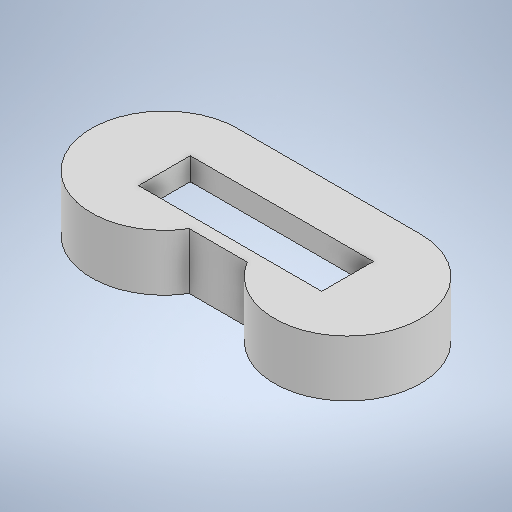
# Autodesk Inventor part: controller_back_v9_d1
Saved by Autodesk Inventor 2025.4 (Build 294407000, 407)
## iProperties
Created: 2026-07-22
Part Number: controller_back_v9_d1
Material: Generic
Document SubType Name: Modeling
Designer: Franchesca
Density: 1 g/cm^3
Appearance: Default
Author: Franchesca
## iProperties of the stored document con_v8_d1_back_3DPrint.ipt
Created: 2026-07-22
Part Number: con_v8_d1_back_3DPrint
Material: Generic
Document SubType Name: Modeling
Designer: Franchesca
Density: 1 g/cm^3
Appearance: Default
Author: Franchesca
Autodesk Inventor part; units mm, degrees
ref_plane "YZ Plane" through (0, 0, 0) normal (1, 0, 0) x (0, 1, 0)
ref_plane "XZ Plane" through (0, 0, 0) normal (0, 1, 0) x (-1, 0, 0)
ref_plane "XY Plane" through (0, 0, 0) normal (0, 0, 1) x (1, 0, 0)
sketch "Sketch1" plane through (0, 0, 0) normal (0, 1, 0) x (-1, 0, 0)
  line L0 (0, 0) -> (0, -22.1379) construction
  line L1 (0, 0) -> (0, 22.1379) construction
  line L2 (0, 0) -> (40.725, 0) construction
  line L3 (0, 0) -> (-40.725, 0) construction
  circle A0 centre (-40.725, 0) radius 30 construction
  circle A1 centre (-40.725, 0) radius 32.5 construction
  circle A2 centre (40.725, 0) radius 30 construction
  circle A3 centre (40.725, 0) radius 32.5 construction
  line L4 (40.725, -30) -> (40.725, 30) construction
  line L5 (40.725, -30) -> (40.725, -32.5) construction
  line L6 (40.725, 30) -> (40.725, 32.5) construction
  line L7 (-40.725, 30) -> (-40.725, -30) construction
  line L8 (-40.725, -32.5) -> (-40.725, -30) construction
  line L9 (-40.725, 30) -> (-40.725, 32.5) construction
  line L10 (40.725, -32.5) -> (-40.725, -32.5) construction
  line L11 (40.725, -30) -> (-40.725, -30) construction
  line L12 (40.725, 32.5) -> (40.725, 14.2758) construction
  line L13 (40.725, 14.2758) -> (-40.725, 14.2758) construction
  line L14 (40.725, 32.5) -> (40.725, 16.7758) construction
  line L15 (40.725, 16.7758) -> (-40.725, 16.7758) construction
  arc A4 (40.725, -30) -> (70.725, 0) centre (40.725, 0) ccw
  arc A5 (70.725, 0) -> (40.725, 30) centre (40.725, 0) ccw
  arc A6 (40.725, 32.5) -> (12.8894, 16.7758) centre (40.725, 0) ccw
  arc A7 (73.225, 0) -> (40.725, 32.5) centre (40.725, 0) ccw
  arc A8 (40.725, -32.5) -> (73.225, 0) centre (40.725, 0) ccw
  line L16 (40.725, -30) -> (-40.725, -30)
  line L17 (-40.725, -32.5) -> (40.725, -32.5)
  line L18 (12.8894, 16.7758) -> (-12.8894, 16.7758)
  line L19 (14.3394, 14.2758) -> (-14.3394, 14.2758)
  arc A9 (40.725, 30) -> (14.3394, 14.2758) centre (40.725, 0) ccw
  arc A10 (-12.8894, 16.7758) -> (-40.725, 32.5) centre (-40.725, 0) ccw
  arc A11 (-14.3394, 14.2758) -> (-40.725, 30) centre (-40.725, 0) ccw
  arc A12 (-40.725, 30) -> (-70.725, 0) centre (-40.725, 0) ccw
  arc A13 (-40.725, 32.5) -> (-73.225, 0) centre (-40.725, 0) ccw
  arc A14 (-70.725, 0) -> (-40.725, -30) centre (-40.725, 0) ccw
  arc A15 (-73.225, 0) -> (-40.725, -32.5) centre (-40.725, 0) ccw
  line L20 (0, 0) -> (39, 0) construction
  line L21 (0, 0) -> (-39, 0) construction
  line L22 (40.725, 0) -> (40.725, -11.5) construction
  line L23 (40.725, 0) -> (40.725, 11.5) construction
  line L24 (-40.725, 0) -> (-40.725, -11.5) construction
  line L25 (-40.725, 0) -> (-40.725, 11.5) construction
  line L26 (40.725, -11.5) -> (-40.725, -11.5)
  line L27 (40.725, 11.5) -> (-40.725, 11.5)
  line L28 (-40.725, 11.5) -> (-40.725, -11.5)
  line L29 (40.725, -11.5) -> (40.725, 11.5)
  dimension "d0" = 22.1379
  dimension "d1" = 22.1379
  dimension "d2" = 40.725
  dimension "d3" = 40.725
  dimension "d4" = 60
  dimension "d5" = 65
  dimension "d6" = 60
  dimension "d7" = 65
  dimension "d8" = 18.2242
  dimension "d9" = 15.7241
  dimension "d10" = 39
  dimension "d11" = 39
  dimension "d12" = 11.5
  dimension "d13" = 11.5
  dimension "d14" = 11.5
  dimension "d15" = 11.5
  constraints: 60 end point, 43 point on circle, 17 point on line, 16 centre point, 11 tangent, 9 concentric, 5 perpendicular, 4 coincident, 3 collinear, 3 vertical, 2 horizontal
  measures "d0" distance of L0.start L0.end
  measures "d1" distance of L0.start L1.end
  measures "d2" distance of L0.start L2.end
  measures "d3" distance of L0.start L3.end
  measures "d4" diameter of A0
  measures "d5" diameter of A1
  measures "d6" diameter of A2
  measures "d7" diameter of A3
  measures "d8" distance of L6.end L12.end
  measures "d9" distance of L6.end L14.end
  measures "d10" distance of L0.start L20.end
  measures "d11" distance of L0.start L21.end
  measures "d12" distance of L22.start L22.end
  measures "d13" distance of L22.start L23.end
  measures "d14" distance of L24.start L24.end
  measures "d15" distance of L24.start L25.end
extrude "Extrusion1" add sketch "Sketch1" against normal blind 10 contours L16 A14 A12 A11 L19 A9 A5 A4
extrude "Extrusion2" add sketch "Sketch1" against normal blind 25 contours A7 A8 L17 A15 A13 A10 L18 A6
ref_plane "Work Plane1" through (0, -25, 0) normal (0, -1, 0) x (1, 0, 0)
body "Solid1"
